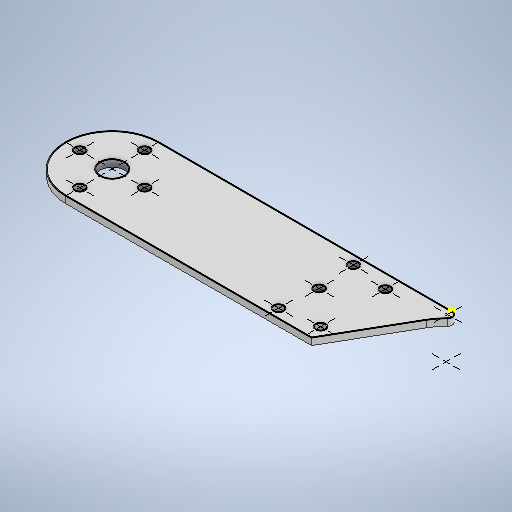
# Autodesk Inventor part: CAM_axis_2_4_connector_frame_powered
Saved by Autodesk Inventor 2025.2 (Build 292293000, 293)
## iProperties
Created: 2025-08-09
Part Number: CAM_axis_2_4_connector_frame_powered
Material: Generic
Document SubType Name: Modeling
Designer: User
Density: 1 g/cm^3
Appearance: Default
Author: User
Autodesk Inventor part; units mm, degrees
ref_plane "YZ Plane" through (0, 0, 0) normal (1, 0, 0) x (0, 1, 0)
ref_plane "XZ Plane" through (0, 0, 0) normal (0, 1, 0) x (-1, 0, 0)
ref_plane "XY Plane" through (0, 0, 0) normal (0, 0, 1) x (1, 0, 0)
sketch "Sketch1" plane through (0, 0, 0) normal (0, 1, 0) x (-1, 0, 0)
  circle A0 centre (19.4253, 18.07) radius 1.05
  circle A1 centre (11.4453, 17) radius 1.05
  circle A2 centre (18.7453, 10) radius 1.05
  circle A3 centre (11.4453, 3) radius 1.05
  circle A4 centre (19.4253, 1.93) radius 1.05
  circle A5 centre (63.4253, 10) radius 2.6
  circle A6 centre (63.4253, 17) radius 1.05
  circle A7 centre (56.4253, 10) radius 1.05
  circle A8 centre (63.4253, 3) radius 1.05
  circle A9 centre (70.4253, 10) radius 1.05
  line L0 (10.3779, 20) -> (1.2846, 4.25)
  arc A10 (-0.694, 1.72) -> (1.2846, 4.25) centre (-8.6747, 10) ccw
  arc A11 (-0.694, 1.72) -> (0, 0) centre (0, 1) ccw
  line L1 (63.4253, 0) -> (0, 0)
  arc A12 (63.4253, 0) -> (63.4253, 20) centre (63.4253, 10) ccw
  line L2 (10.3779, 20) -> (63.4253, 20)
  point P0 (0, 0)
  constraints: 13 centre point, 8 equal radius, 6 end point, 6 point on circle, 5 tangent, 2 horizontal, 1 parallel, 33 other
extrude "Extrusion1" add sketch "Sketch1" against normal blind 1.5
body "Solid1"
